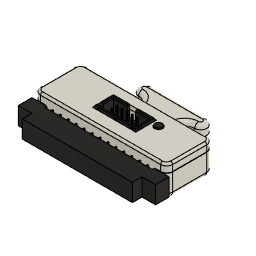
SpeedDOS_ParUP v5 (Autodesk Fusion 360 design; units mm, degrees)
Autodesk Fusion 360 part; units mm, degrees
sketch "UP-PAR-Adaptor" plane through (0, 0, 0) normal (0, 0, 1) x (1, 0, 0) in component "PCB"
  line L0 (54, 20) -> (0, 20)
  line L1 (0, 0) -> (54, 0)
  line L2 (54, 0) -> (54, 20)
  line L3 (0, 20) -> (0, 0)
  line L4 (1.3215, 4.5593) -> (1.3215, 2.9337)
  line L5 (2.4331, 2.9337) -> (3.3362, 2.9337)
  arc A0 (3.3362, 4.1529) -> (2.9298, 4.5593) centre (2.9298, 4.1529) ccw
  arc A1 (2.9298, 4.5593) -> (2.4331, 4.1981) centre (2.9298, 4.0372) ccw
  line L6 (0.87, 4.1981) -> (1.3215, 4.5593)
  line L7 (0.87, 2.9337) -> (1.7731, 2.9337)
  arc A2 (3.2007, 3.8368) -> (3.3362, 4.1529) centre (2.8997, 4.1529) ccw
  line L8 (3.2007, 3.8368) -> (2.4331, 2.9337)
  line L9 (39.6875, 9.2075) -> (39.6875, 6.6675)
  line L10 (43.09, -1) -> (43.09, 0)
  line L11 (46.55, 0) -> (46.55, -1)
  line L12 (51.01, -1) -> (51.01, 0)
  line L13 (13.97, 8.89) -> (16.51, 8.89)
  line L14 (51.01, 0) -> (50.51, 0)
  circle A3 centre (5, 15) radius 3.1789
  line L15 (50.51, 0) -> (50.51, -1)
  line L16 (39.6875, 9.2075) -> (44.7675, 9.2075)
  line L17 (45.82, 0.1) -> (45.82, -1)
  line L18 (16.51, 13.97) -> (16.51, 8.89)
  line L19 (16.51, 13.97) -> (13.97, 13.97)
  line L20 (43.09, 0) -> (42.59, 0)
  circle A4 centre (5, 15) radius 1.7463
  circle A5 centre (49, 15) radius 3.1789
  line L21 (44.7675, 6.6675) -> (39.6875, 6.6675)
  circle A6 centre (49, 15) radius 1.7463
  line L22 (49.78, 0.1) -> (49.78, -1)
  line L23 (43.82, 0.1) -> (43.82, -1)
  line L24 (7.45, -1) -> (7.45, 0)
  line L25 (3.49, 0) -> (2.99, 0)
  line L26 (37.9, 0.1) -> (37.9, -1)
  line L27 (24.02, 0.1) -> (24.02, -1)
  line L28 (34.67, 0) -> (34.67, -1)
  line L29 (22.79, 0) -> (22.79, -1)
  line L30 (13.97, 8.89) -> (13.97, 13.97)
  line L31 (44.7675, 6.6675) -> (44.7675, 9.2075)
  line L32 (23.29, 0) -> (22.79, 0)
  line L33 (29.98, 0.1) -> (29.98, -1)
  line L34 (38.63, 0) -> (38.63, -1)
  line L35 (35.17, -1) -> (35.17, 0)
  line L36 (27.25, 0) -> (26.75, 0)
  line L37 (26.75, 0) -> (26.75, -1)
  line L38 (35.17, 0) -> (34.67, 0)
  line L39 (47.05, -1) -> (47.05, 0)
  line L40 (33.94, 0.1) -> (33.94, -1)
  line L41 (23.29, -1) -> (23.29, 0)
  line L42 (47.05, 0) -> (46.55, 0)
  line L43 (27.98, 0.1) -> (27.98, -1)
  line L44 (42.59, 0) -> (42.59, -1)
  line L45 (41.86, 0.1) -> (41.86, -1)
  line L46 (35.9, 0.1) -> (35.9, -1)
  line L47 (30.71, 0) -> (30.71, -1)
  line L48 (27.25, -1) -> (27.25, 0)
  line L49 (31.94, 0.1) -> (31.94, -1)
  line L50 (39.86, 0.1) -> (39.86, -1)
  line L51 (26.02, 0.1) -> (26.02, -1)
  line L52 (39.13, 0) -> (38.63, 0)
  line L53 (47.78, 0.1) -> (47.78, -1)
  line L54 (31.21, 0) -> (30.71, 0)
  line L55 (10.18, 0.1) -> (10.18, -1)
  line L56 (7.45, 0) -> (6.95, 0)
  line L57 (8.18, 0.1) -> (8.18, -1)
  line L58 (6.22, 0.1) -> (6.22, -1)
  line L59 (4.22, 0.1) -> (4.22, -1)
  line L60 (3.49, -1) -> (3.49, 0)
  line L61 (39.13, -1) -> (39.13, 0)
  line L62 (31.21, -1) -> (31.21, 0)
  line L63 (53.8, -1) -> (0.2, -1)
  line L64 (6.95, 0) -> (6.95, -1)
  line L65 (0.2, -1) -> (0.2, 0)
  line L66 (0.2, 0) -> (-2.3, 0)
  line L67 (14.14, 0.1) -> (14.14, -1)
  line L68 (2.99, 0) -> (2.99, -1)
  line L69 (-7.25, 0) -> (-7.25, -6.8)
  line L70 (-2.3, 0) -> (-4, 0)
  line L71 (61.25, 0) -> (61.25, -6.8)
  line L72 (58, 0) -> (56.3, 0)
  line L73 (59.7, 0) -> (58, 0)
  line L74 (18.83, 0) -> (18.83, -1)
  line L75 (14.87, 0) -> (14.87, -1)
  line L76 (20.06, 0.1) -> (20.06, -1)
  line L77 (22.06, 0.1) -> (22.06, -1)
  line L78 (19.33, -1) -> (19.33, 0)
  line L79 (56.3, -1.6) -> (56.3, 0)
  line L80 (35.89, 15.3338) -> (35.89, 10.2537)
  line L81 (18.1, 0.1) -> (18.1, -1)
  line L82 (37.16, 8.825) -> (37.16, 7.3962)
  line L83 (16.84, 8.825) -> (16.84, 10.2537)
  line L84 (-4, 0) -> (-5.7, 0)
  line L85 (56.3, -6.8) -> (56.3, -5.2)
  line L86 (-2.3, -1.6) -> (-2.3, 0)
  line L87 (37.16, 7.3962) -> (16.84, 7.3962)
  line L88 (-5.7, -4.2) -> (-5.7, -2.6)
  line L89 (58, -7.2333) -> (58, -4.3667)
  line L90 (16.84, 7.3962) -> (16.84, 8.825)
  line L91 (16.1, 0.1) -> (16.1, -1)
  line L92 (-4, -8.7333) -> (-4, -11.6)
  line L93 (-5.7, -6.8) -> (-7.25, -6.8)
  line L94 (15.37, -1) -> (15.37, 0)
  line L95 (19.33, 0) -> (18.83, 0)
  line L96 (58, -8.052) -> (58, -7.9147)
  line L97 (-2.3, -4.2) -> (-2.3, -2.6)
  line L98 (-5.7, -6.8) -> (-5.7, -5.2)
  line L99 (18.11, 10.2537) -> (18.11, 15.3338)
  line L100 (12.14, 0.1) -> (12.14, -1)
  line L101 (59.7, -1.6) -> (59.7, 0)
  line L102 (15.37, 0) -> (14.87, 0)
  line L103 (29.0638, 16.6038) -> (37.16, 16.6038)
  line L104 (18.11, 15.3338) -> (24.9362, 15.3338)
  line L105 (16.84, 10.2537) -> (16.84, 16.6038)
  line L106 (-2.3, -6.8) -> (-2.3, -5.2)
  line L107 (10.91, 0) -> (10.91, -1)
  line L108 (24.9362, 16.6038) -> (29.0638, 16.6038)
  line L109 (11.41, -1) -> (11.41, 0)
  line L110 (24.9362, 15.3338) -> (29.0638, 15.3338)
  line L111 (56.3, -6.8) -> (54.5, -6.8)
  line L112 (11.41, 0) -> (10.91, 0)
  line L113 (-4, -4.3667) -> (-4, -7.2333)
  line L114 (59.7, -6.8) -> (59.7, -5.2)
  line L115 (37.16, 10.2537) -> (37.16, 8.825)
  line L116 (56.3, -4.2) -> (56.3, -2.6)
  line L117 (16.84, 16.6038) -> (24.9362, 16.6038)
  line L118 (-2.3, -6.8) -> (-5.7, -6.8)
  line L119 (54.5, -11.6) -> (-0.5, -11.6)
  line L120 (35.89, 8.6662) -> (18.11, 8.6662)
  line L121 (29.0638, 15.3338) -> (35.89, 15.3338)
  line L122 (35.89, 8.825) -> (35.89, 8.6662)
  line L123 (58, -2.8667) -> (58, 0)
  line L124 (-4, -3.548) -> (-4, -3.6853)
  line L125 (58, -3.6853) -> (58, -3.548)
  line L126 (-5.7, -1.6) -> (-5.7, 0)
  line L127 (17.6337, 10.2537) -> (16.84, 10.2537)
  line L128 (59.7, -4.2) -> (59.7, -2.6)
  line L129 (-4, -7.9147) -> (-4, -8.052)
  line L130 (58, -11.6) -> (58, -8.7333)
  line L131 (32.08, 14.6987) -> (32.3975, 15.0162)
  line L132 (61.25, 0) -> (59.7, 0)
  line L133 (36.3663, 8.19) -> (17.6337, 8.19)
  line L134 (36.3663, 8.19) -> (35.89, 8.6662)
  line L135 (35.89, 8.825) -> (36.3663, 8.825)
  line L136 (35.89, 10.2537) -> (36.3663, 10.2537)
  arc A7 (26.5238, 7.3962) -> (27.635, 7.3962) centre (27.0794, 7.3962) ccw
  line L137 (18.11, 8.6662) -> (17.6337, 8.19)
  line L138 (59.7, -6.8) -> (56.3, -6.8)
  line L139 (53.8, 0) -> (53.8, -1)
  line L140 (32.715, 15.0162) -> (32.5563, 15.0162)
  line L141 (32.5563, 15.0162) -> (32.3975, 15.0162)
  line L142 (31.9213, 15.0162) -> (32.08, 14.8575)
  line L143 (36.3663, 8.825) -> (37.16, 8.825)
  line L144 (36.3663, 8.19) -> (36.3663, 8.825)
  line L145 (24.9362, 15.3338) -> (24.9362, 15.81)
  line L146 (31.9213, 15.0162) -> (31.7625, 15.0162)
  line L147 (56.3, 0) -> (53.8, 0)
  line L148 (-4, 0) -> (-4, -2.8667)
  line L149 (24.9362, 15.81) -> (24.9362, 16.6038)
  line L150 (31.7625, 15.0162) -> (32.08, 14.6987)
  line L151 (18.11, 10.2537) -> (17.6337, 10.2537)
  line L152 (31.7625, 15.0162) -> (31.6038, 15.0162)
  line L153 (29.0638, 15.81) -> (36.3663, 15.81)
  line L154 (32.08, 14.54) -> (32.5563, 15.0162)
  line L155 (29.0638, 15.3338) -> (29.0638, 15.81)
  line L156 (18.11, 8.825) -> (18.11, 10.2537)
  line L157 (54.5, -6.8) -> (54.5, -11.6)
  line L158 (31.6038, 15.0162) -> (32.08, 14.54)
  line L159 (31.445, 15.0162) -> (32.08, 14.3812)
  line L160 (36.3663, 15.81) -> (35.89, 15.3338)
  line L161 (35.89, 10.2537) -> (35.89, 8.825)
  line L162 (-5.7, 0) -> (-7.25, 0)
  line L163 (18.11, 15.3338) -> (17.6337, 15.81)
  line L164 (-0.5, -11.6) -> (-0.5, -6.8)
  line L165 (17.6337, 8.825) -> (16.84, 8.825)
  arc A8 (18.11, 7.3962) -> (19.38, 7.3962) centre (18.745, 7.3962) ccw
  arc A9 (34.62, 7.3962) -> (35.89, 7.3962) centre (35.255, 7.3962) ccw
  line L166 (29.0638, 15.81) -> (29.0638, 16.6038)
  line L167 (-0.5, -6.8) -> (-2.3, -6.8)
  line L168 (32.08, 14.8575) -> (32.2388, 15.0162)
  line L169 (32.2388, 15.0162) -> (31.9213, 15.0162)
  line L170 (61.25, -6.8) -> (59.7, -6.8)
  line L171 (18.11, 8.6662) -> (18.11, 8.825)
  line L172 (37.16, 16.6038) -> (37.16, 10.2537)
  line L173 (31.6038, 15.0162) -> (31.445, 15.0162)
  arc A10 (39.25, 12.55) -> (38.45, 12.55) centre (38.85, 12.85) ccw
  arc A11 (38.45, 17.45) -> (39.2, 17.5) centre (38.8467, 17.1498) ccw
  line L174 (17.6337, 10.2537) -> (17.6337, 15.81)
  circle A12 centre (41, 15) radius 1.75
  line L175 (32.08, 14.3812) -> (32.715, 15.0162)
  line L176 (32.3975, 15.0162) -> (32.2388, 15.0162)
  line L177 (42.45, 12) -> (39.6, 12)
  line L178 (39.55, 18) -> (42.45, 18)
  arc A13 (43.55, 12.55) -> (42.8, 12.5) centre (43.1533, 12.8502) ccw
  line L179 (36.3663, 10.2537) -> (36.3663, 15.81)
  line L180 (18.11, 8.825) -> (17.6337, 8.825)
  line L181 (44, 17.75) -> (44, 12.25)
  arc A14 (42.75, 17.45) -> (43.5, 17.5) centre (43.1467, 17.1498) ccw
  line L182 (36.3663, 10.2537) -> (37.16, 10.2537)
  circle A15 centre (41, 15) radius 1.4
  line L183 (38, 12.6) -> (38, 17.75)
  line L184 (24.9362, 15.81) -> (17.6337, 15.81)
  line L185 (17.6337, 8.825) -> (17.6337, 8.19)
  line L186 (49.78, 0.1) -> (49.78, 4)
  line L187 (49.28, 3) -> (49.28, 2)
  arc A16 (44.32, 2) -> (45.32, 2) centre (44.82, 2) ccw
  line L188 (45.82, 0.1) -> (45.82, 4)
  line L189 (45.32, 3) -> (45.32, 2)
  arc A17 (45.32, 3) -> (44.32, 3) centre (44.82, 3) ccw
  arc A18 (49.78, 4) -> (47.78, 4) centre (48.78, 4) ccw
  arc A19 (49.28, 3) -> (48.28, 3) centre (48.78, 3) ccw
  line L190 (47.78, 0.1) -> (47.78, 4)
  arc A20 (45.82, 4) -> (43.82, 4) centre (44.82, 4) ccw
  line L191 (44.32, 3) -> (44.32, 2)
  line L192 (20.56, 3) -> (20.56, 2)
  arc A21 (17.6, 3) -> (16.6, 3) centre (17.1, 3) ccw
  line L193 (41.86, 0.1) -> (41.86, 4)
  arc A22 (33.44, 3) -> (32.44, 3) centre (32.94, 3) ccw
  line L194 (13.64, 3) -> (13.64, 2)
  arc A23 (6.22, 4) -> (4.22, 4) centre (5.22, 4) ccw
  line L195 (12.14, 0.1) -> (12.14, 4)
  arc A24 (5.72, 3) -> (4.72, 3) centre (5.22, 3) ccw
  arc A25 (26.02, 4) -> (24.02, 4) centre (25.02, 4) ccw
  arc A26 (36.4, 2) -> (37.4, 2) centre (36.9, 2) ccw
  arc A27 (48.28, 2) -> (49.28, 2) centre (48.78, 2) ccw
  arc A28 (24.52, 2) -> (25.52, 2) centre (25.02, 2) ccw
  line L196 (39.86, 0.1) -> (39.86, 4)
  arc A29 (28.48, 2) -> (29.48, 2) centre (28.98, 2) ccw
  arc A30 (16.6, 2) -> (17.6, 2) centre (17.1, 2) ccw
  arc A31 (10.18, 4) -> (8.18, 4) centre (9.18, 4) ccw
  line L197 (24.52, 3) -> (24.52, 2)
  arc A32 (18.1, 4) -> (16.1, 4) centre (17.1, 4) ccw
  arc A33 (13.64, 3) -> (12.64, 3) centre (13.14, 3) ccw
  arc A34 (9.68, 3) -> (8.68, 3) centre (9.18, 3) ccw
  arc A35 (33.94, 4) -> (31.94, 4) centre (32.94, 4) ccw
  arc A36 (41.86, 4) -> (39.86, 4) centre (40.86, 4) ccw
  line L198 (33.94, 0.1) -> (33.94, 4)
  arc A37 (20.56, 2) -> (21.56, 2) centre (21.06, 2) ccw
  line L199 (35.9, 0.1) -> (35.9, 4)
  line L200 (29.98, 0.1) -> (29.98, 4)
  line L201 (33.44, 3) -> (33.44, 2)
  line L202 (41.36, 3) -> (41.36, 2)
  arc A38 (4.72, 2) -> (5.72, 2) centre (5.22, 2) ccw
  line L203 (5.72, 3) -> (5.72, 2)
  line L204 (9.68, 3) -> (9.68, 2)
  line L205 (21.56, 3) -> (21.56, 2)
  line L206 (36.4, 3) -> (36.4, 2)
  line L207 (12.64, 3) -> (12.64, 2)
  line L208 (4.22, 0.1) -> (4.22, 4)
  line L209 (48.28, 3) -> (48.28, 2)
  arc A39 (8.68, 2) -> (9.68, 2) centre (9.18, 2) ccw
  line L210 (17.6, 3) -> (17.6, 2)
  arc A40 (22.06, 4) -> (20.06, 4) centre (21.06, 4) ccw
  arc A41 (41.36, 3) -> (40.36, 3) centre (40.86, 3) ccw
  line L211 (37.9, 0.1) -> (37.9, 4)
  line L212 (32.44, 3) -> (32.44, 2)
  line L213 (31.94, 0.1) -> (31.94, 4)
  line L214 (4.72, 3) -> (4.72, 2)
  arc A42 (37.4, 3) -> (36.4, 3) centre (36.9, 3) ccw
  arc A43 (29.48, 3) -> (28.48, 3) centre (28.98, 3) ccw
  line L215 (16.6, 3) -> (16.6, 2)
  line L216 (20.06, 0.1) -> (20.06, 4)
  arc A44 (40.36, 2) -> (41.36, 2) centre (40.86, 2) ccw
  line L217 (27.98, 0.1) -> (27.98, 4)
  line L218 (26.02, 0.1) -> (26.02, 4)
  line L219 (24.02, 0.1) -> (24.02, 4)
  line L220 (28.48, 3) -> (28.48, 2)
  arc A45 (29.98, 4) -> (27.98, 4) centre (28.98, 4) ccw
  arc A46 (37.9, 4) -> (35.9, 4) centre (36.9, 4) ccw
  line L221 (29.48, 3) -> (29.48, 2)
  line L222 (6.22, 0.1) -> (6.22, 4)
  line L223 (43.82, 0.1) -> (43.82, 4)
  arc A47 (25.52, 3) -> (24.52, 3) centre (25.02, 3) ccw
  arc A48 (32.44, 2) -> (33.44, 2) centre (32.94, 2) ccw
  line L224 (25.52, 3) -> (25.52, 2)
  line L225 (22.06, 0.1) -> (22.06, 4)
  line L226 (37.4, 3) -> (37.4, 2)
  line L227 (40.36, 3) -> (40.36, 2)
  line L228 (38, 12.2) -> (38, 12.6)
  line L229 (24.206, 13.016) -> (24.714, 13.016)
  line L230 (31.826, 10.984) -> (31.826, 10.476)
  line L231 (31.826, 10.476) -> (32.334, 10.476)
  line L232 (31.826, 13.016) -> (32.334, 13.016)
  line L233 (32.334, 13.016) -> (32.334, 13.524)
  arc A49 (43.5, 17.5) -> (42.75, 17.45) centre (43.1467, 17.1498) ccw
  line L234 (24.714, 13.524) -> (24.206, 13.524)
  line L235 (29.286, 10.476) -> (29.794, 10.476)
  line L236 (29.286, 13.524) -> (29.286, 13.016)
  line L237 (31.826, 13.524) -> (31.826, 13.016)
  line L238 (24.206, 10.984) -> (24.206, 10.476)
  arc A50 (43.8, 12) -> (44, 12.2) centre (43.8, 12.2) ccw
  line L239 (26.746, 10.476) -> (27.254, 10.476)
  line L240 (26.746, 13.524) -> (26.746, 13.016)
  line L241 (29.794, 10.984) -> (29.286, 10.984)
  line L242 (42.9, 18.5) -> (42.9, 18)
  line L243 (14.14, 0.1) -> (14.14, 4)
  arc A51 (38.2, 18) -> (38, 17.8) centre (38.2, 17.8) ccw
  line L244 (21.666, 13.016) -> (22.174, 13.016)
  line L245 (38.2, 18) -> (39.55, 18)
  line L246 (21.666, 13.524) -> (21.666, 13.016)
  line L247 (21.666, 10.476) -> (22.174, 10.476)
  line L248 (8.18, 0.1) -> (8.18, 4)
  line L249 (38, 17.75) -> (38, 17.8)
  line L250 (44, 17.8) -> (44, 17.75)
  line L251 (22.174, 13.016) -> (22.174, 13.524)
  line L252 (43.8, 12) -> (42.45, 12)
  arc A52 (42.8, 12.5) -> (43.55, 12.55) centre (43.1533, 12.8502) ccw
  line L253 (27.254, 10.476) -> (27.254, 10.984)
  line L254 (29.794, 13.524) -> (29.286, 13.524)
  line L255 (24.714, 10.984) -> (24.206, 10.984)
  line L256 (24.206, 13.524) -> (24.206, 13.016)
  line L257 (39.6, 12) -> (38.2, 12)
  line L258 (42.45, 18) -> (43.8, 18)
  line L259 (29.794, 13.016) -> (29.794, 13.524)
  line L260 (10.18, 0.1) -> (10.18, 4)
  line L261 (16.1, 0.1) -> (16.1, 4)
  line L262 (32.334, 10.984) -> (31.826, 10.984)
  line L263 (29.286, 10.984) -> (29.286, 10.476)
  arc A53 (12.64, 2) -> (13.64, 2) centre (13.14, 2) ccw
  line L264 (29.794, 10.476) -> (29.794, 10.984)
  line L265 (29.286, 13.016) -> (29.794, 13.016)
  line L266 (8.68, 3) -> (8.68, 2)
  line L267 (32.334, 13.524) -> (31.826, 13.524)
  line L268 (24.714, 13.016) -> (24.714, 13.524)
  arc A54 (39.2, 17.5) -> (38.45, 17.45) centre (38.8467, 17.1498) ccw
  arc A55 (14.14, 4) -> (12.14, 4) centre (13.14, 4) ccw
  line L269 (27.254, 10.984) -> (26.746, 10.984)
  line L270 (42.9, 18) -> (43.6, 18)
  line L271 (24.206, 10.476) -> (24.714, 10.476)
  line L272 (18.1, 0.1) -> (18.1, 4)
  line L273 (44, 12.25) -> (44, 12.2)
  line L274 (26.746, 13.016) -> (27.254, 13.016)
  line L275 (22.174, 10.984) -> (21.666, 10.984)
  line L276 (21.666, 10.984) -> (21.666, 10.476)
  line L277 (26.746, 10.984) -> (26.746, 10.476)
  line L278 (22.174, 10.476) -> (22.174, 10.984)
  arc A56 (44, 17.8) -> (43.8, 18) centre (43.8, 17.8) ccw
  line L279 (24.714, 10.476) -> (24.714, 10.984)
  line L280 (27.254, 13.524) -> (26.746, 13.524)
  arc A57 (38.45, 12.55) -> (39.25, 12.55) centre (38.85, 12.85) ccw
  line L281 (32.334, 10.476) -> (32.334, 10.984)
  arc A58 (21.56, 3) -> (20.56, 3) centre (21.06, 3) ccw
  line L282 (43.6, 11.5) -> (43.6, 12)
  line L283 (27.254, 13.016) -> (27.254, 13.524)
  line L284 (39.1, 12) -> (38.4, 12)
  line L285 (43.6, 12) -> (42.9, 12)
  arc A59 (38, 12.2) -> (38.2, 12) centre (38.2, 12.2) ccw
  line L286 (38.4, 18.5) -> (38.4, 18)
  line L287 (39.1, 18) -> (39.1, 18.5)
  line L288 (42.9, 11.5) -> (43.6, 11.5)
  line L289 (43.6, 18) -> (43.6, 18.5)
  line L290 (39.1, 11.5) -> (39.1, 12)
  line L291 (43.6, 18.5) -> (42.9, 18.5)
  line L292 (38.4, 18) -> (39.1, 18)
  line L293 (42.9, 12) -> (42.9, 11.5)
  line L294 (39.1, 18.5) -> (38.4, 18.5)
  line L295 (38.4, 11.5) -> (39.1, 11.5)
  line L296 (38.4, 12) -> (38.4, 11.5)
  line L297 (22.174, 13.524) -> (21.666, 13.524)
extrude "Extrude1" add sketch "UP-PAR-Adaptor" against normal blind 1.6 contours L0 L1 L2 L3 L14 L17 L20 L22 L23 L25 L26 L27 L32 L33 L36 L38 L40 L42 L43 L45 L46 L49 L50 L51 L52 L53 L54 L55 L56 L57 L58 L59 L66 L67 L76 L77 L81 L91 L95 L100 L102 L112 L147 L186 L188 A18 L190 A20 L193 A23 L195 A25 L196 A31 A32 A35 A36 L198 L199 L200 L208 A40 L211 L213 L216 L217 L218 L219 A45 A46 L222 L223 L225 L243 L248 L260 L261 A55 L272 | L1 L22 L53 L186 A18 L190 | L1 L58 L59 A23 L208 L222 | L1 L17 L23 L188 A20 L223 | L1 L55 L57 A31 L248 L260 | L1 L45 L50 L193 L196 A36 | L1 L67 L100 L195 L243 A55 | L1 L26 L46 L199 L211 A46 | L1 L81 L91 A32 L261 L272 | L1 L40 L49 A35 L198 L213 | L1 L76 L77 A40 L216 L225 | L1 L33 L43 L200 L217 A45 | L1 L27 L51 A25 L218 L219 | L9 L16 L21 L31 | L13 L18 L19 L30 | A3 | A5 | L80 L136 L160 L179 | L80 L99 L104 L110 L120 L121 L122 L156 L161 L171 | L121 L153 L155 L160 | L115 L135 L136 L143 L161 L182 | L108 L110 L145 L149 L155 L166 | L103 L153 L166 L172 L179 L182 | L122 L134 L135 L144 | L104 L145 L163 L184 | L120 L133 L134 L137 | L82 L87 L90 L133 L143 L144 L165 L185 | L99 L151 L163 L174 | L105 L117 L127 L149 L174 L184 | L137 L171 L180 L185 | L83 L127 L151 L156 L165 L180 | L87 A9 | L87 A7 | L87 A8 | L131 L142 L146 L150 L168 L176 | L131 L141 L150 L152 L154 L158 | L140 L154 L158 L159 L173 L175 | L142 L168 L169 | A10 A57 | A11 A54 | A12 | L177 L178 L181 L183 L228 A50 A51 L245 L249 L250 L252 L257 L258 L270 L273 A56 L284 L285 A59 L292 | L252 L282 L285 L288 L293 | L257 L284 L290 L295 L296 | L242 L258 L270 L289 L291 | L245 L286 L287 L292 L294 | A13 A52 | A14 A49 | A15 | L187 A19 A27 L209 | A16 L189 A17 L191 | L192 A37 L205 A58 | A21 A30 L210 L215 | A22 L201 L212 A48 | L194 A33 L207 A53 | A24 A38 L203 L214 | A26 L206 A42 L226 | A28 L197 A47 L224 | A29 A43 L220 L221 | A34 L204 A39 L266 | L202 A41 A44 L227 | L229 L234 L256 L268 | L230 L231 L262 L281 | L232 L233 L237 L267 | L235 L241 L263 L264 | L236 L254 L259 L265 | L238 L255 L271 L279 | L239 L253 L269 L277 | L240 L274 L280 L283 | L244 L246 L251 L297 | L247 L275 L276 L278 makes body 1 in component "PCB"
extrude "Extrude2" add sketch "UP-PAR-Adaptor" along normal blind 3 contours L177 L178 L181 L183 L228 A50 A51 L245 L249 L250 L252 L257 L258 L270 L273 A56 L284 L285 A59 L292 bodies 1 in component "PCB"
extrude "Extrude3" add sketch "UP-PAR-Adaptor" along normal blind 3.8 contours A10 A57 | A11 A54 | A13 A52 | A14 A49 bodies 1 in component "PCB"
extrude "Extrude4" add sketch "UP-PAR-Adaptor" along normal blind 9 contours A12 | A15 bodies 1 in component "PCB"
extrude "Extrude5" add sketch "UP-PAR-Adaptor" along normal blind 2.3 contours L80 L99 L104 L110 L120 L121 L122 L156 L161 L171 | L115 L135 L136 L143 L161 L182 | L108 L110 L145 L149 L155 L166 | L83 L127 L151 L156 L165 L180 bodies 1 in component "PCB"
extrude "Extrude6" add sketch "UP-PAR-Adaptor" along normal blind 9.3 contours L80 L136 L160 L179 | L121 L153 L155 L160 | L103 L153 L166 L172 L179 L182 | L122 L134 L135 L144 | L104 L145 L163 L184 | L120 L133 L134 L137 | L82 L87 L90 L133 L143 L144 L165 L185 | L99 L151 L163 L174 | L105 L117 L127 L149 L174 L184 | L137 L171 L180 L185 bodies 1 in component "PCB"
extrude "Extrude7" add sketch "UP-PAR-Adaptor" along normal blind 8.8 contours L229 L234 L256 L268 | L230 L231 L262 L281 | L232 L233 L237 L267 | L235 L241 L263 L264 | L236 L254 L259 L265 | L238 L255 L271 L279 | L239 L253 L269 L277 | L240 L274 L280 L283 | L244 L246 L251 L297 | L247 L275 L276 L278 bodies 1 in component "PCB"
extrude "Extrude8" add sketch "UP-PAR-Adaptor" along normal blind 8.8 contours L87 A9 | L87 A7 | L87 A8 bodies 1 in component "PCB"
extrude "Extrude9" add sketch "UP-PAR-Adaptor" along normal blind 4.3 and the other way blind 4.4 contours L1 L63 L65 L66 L69 L70 L71 L72 L73 L84 L93 L111 L118 L119 L132 L138 L139 L147 L157 L162 L164 L167 L170 | L1 L12 L14 L15 L63 | L1 L25 L60 L63 L68 | L1 L11 L39 L42 L63 | L1 L24 L56 L63 L64 | L1 L10 L20 L44 L63 | L1 L63 L107 L109 L112 | L1 L34 L52 L61 L63 | L1 L63 L75 L94 L102 | L1 L28 L35 L38 L63 | L1 L63 L74 L78 L95 | L1 L47 L54 L62 L63 | L1 L29 L32 L41 L63 | L1 L36 L37 L48 L63 bodies 1 in component "PCB"
extrude "Extrude10" add sketch "UP-PAR-Adaptor" along normal blind 0.5 contours L1 L22 L53 L63 | L1 L22 L53 L186 A18 L190 | L1 L58 L59 A23 L208 L222 | L1 L58 L59 L63 | L1 L17 L23 L63 | L1 L17 L23 L188 A20 L223 | L1 L55 L57 A31 L248 L260 | L1 L55 L57 L63 | L1 L45 L50 L63 | L1 L45 L50 L193 L196 A36 | L1 L67 L100 L195 L243 A55 | L1 L63 L67 L100 | L1 L26 L46 L63 | L1 L26 L46 L199 L211 A46 | L1 L81 L91 A32 L261 L272 | L1 L63 L81 L91 | L1 L40 L49 L63 | L1 L40 L49 A35 L198 L213 | L1 L76 L77 A40 L216 L225 | L1 L63 L76 L77 | L1 L33 L43 L63 | L1 L33 L43 L200 L217 A45 | L1 L27 L51 A25 L218 L219 | L1 L27 L51 L63 bodies 1 in component "PCB"
extrude "Extrude11" add sketch "UP-PAR-Adaptor" against normal blind 0.5 from surface at -1.6 contours L1 L22 L53 L63 | L1 L22 L53 L186 A18 L190 | L1 L58 L59 A23 L208 L222 | L1 L58 L59 L63 | L1 L17 L23 L63 | L1 L17 L23 L188 A20 L223 | L1 L55 L57 A31 L248 L260 | L1 L55 L57 L63 | L1 L45 L50 L63 | L1 L45 L50 L193 L196 A36 | L1 L67 L100 L195 L243 A55 | L1 L63 L67 L100 | L1 L26 L46 L63 | L1 L26 L46 L199 L211 A46 | L1 L81 L91 A32 L261 L272 | L1 L63 L81 L91 | L1 L40 L49 L63 | L1 L40 L49 A35 L198 L213 | L1 L76 L77 A40 L216 L225 | L1 L63 L76 L77 | L1 L33 L43 L63 | L1 L33 L43 L200 L217 A45 | L1 L27 L51 A25 L218 L219 | L1 L27 L51 L63 bodies 1 in component "PCB"
chamfer "Chamfer1" distance 0.5 angle 45 7 edges at (27, 8.6662, 9.3) (35.89, 12.7938, 9.3) (32.4769, 15.3338, 9.3) (21.5231, 15.3338, 9.3) (18.11, 12.7938, 9.3) (18.11, 8.7456, 9.3) (35.89, 8.7456, 9.3) on bodies 1 in component "PCB"
ref_plane "WorkPlane1" through (0, 0, -4.4) normal (0, 0, 1) x (1, 0, 0) in component "bottom_shell"
sketch "bottom" plane through (0, 0, -4.4) normal (0, 0, 1) x (1, 0, 0) in component "bottom_shell"
  circle A0 centre (49, 15) radius 1.7463 construction
  line L0 (54, 0) -> (54, 20) construction
  line L1 (54, 20) -> (0, 20) construction
  line L2 (0, 20) -> (0, 0) construction
  circle A1 centre (5, 15) radius 1.7463 construction
  line L3 (27, 20) -> (27, -5) construction
  line L4 (54, 0) -> (0, 0) construction
  circle A2 centre (49, 15) radius 1.75
  circle A3 centre (5, 15) radius 1.75
  line L5 (60, 3) -> (60, 20)
  line L6 (-6, 3) -> (-6, 20)
  line L7 (57, 23) -> (-3, 23)
  line L8 (57, 0) -> (-3, 0)
  arc A4 (57, 0) -> (60, 3) centre (57, 3) ccw
  arc A5 (60, 20) -> (57, 23) centre (57, 20) ccw
  arc A6 (-3, 23) -> (-6, 20) centre (-3, 20) ccw
  arc A7 (-6, 3) -> (-3, 0) centre (-3, 3) ccw
  line L9 (57, 21) -> (-3, 21)
  arc A8 (-3, 21) -> (-4, 20) centre (-3, 20) ccw
  line L10 (-4, 3) -> (-4, 20)
  arc A9 (-4, 3) -> (-3, 2) centre (-3, 3) ccw
  line L11 (57, 2) -> (-3, 2)
  arc A10 (57, 2) -> (58, 3) centre (57, 3) ccw
  line L12 (58, 3) -> (58, 20)
  arc A11 (58, 20) -> (57, 21) centre (57, 20) ccw
  circle A12 centre (49, 15) radius 4.25
  circle A13 centre (5, 15) radius 4.25
  line L13 (54.6, 1.2) -> (54.6, 2)
  line L14 (-0.6, 0) -> (-0.6, 2)
  circle A14 centre (49, 15) radius 3
  circle A15 centre (5, 15) radius 3
  line L15 (57, 21.8) -> (-3, 21.8)
  arc A16 (-3, 21.8) -> (-4.8, 20) centre (-3, 20) ccw
  line L16 (-4.8, 3) -> (-4.8, 20)
  arc A17 (-4.8, 3) -> (-3, 1.2) centre (-3, 3) ccw
  arc A18 (57, 1.2) -> (58.8, 3) centre (57, 3) ccw
  line L17 (58.8, 3) -> (58.8, 20)
  arc A19 (58.8, 20) -> (57, 21.8) centre (57, 20) ccw
  line L18 (57, 1.2) -> (54.6, 1.2)
  line L19 (-0.6, 1.2) -> (-3, 1.2)
  line L20 (54.6, 1.2) -> (54.6, 0)
  line L21 (41, 28) -> (41, 33) construction
  line L22 (41, 33) -> (13, 33) construction
  line L23 (41, 33) -> (41, 39.5) construction
  line L24 (13, 39) -> (41, 39)
  line L25 (13, 36) -> (13, 39) construction
  arc A20 (13, 39) -> (13, 33) centre (13, 36) ccw
  arc A21 (41, 33) -> (41, 39) centre (41, 36) ccw
  arc A22 (41, 33) -> (41, 23) centre (41, 28) ccw
  arc A23 (13, 23) -> (13, 33) centre (13, 28) ccw
  point P0 (51.01, 0)
  point P1 (60, 0)
  point P2 (60, 23)
  point P3 (-6, 0)
  point P4 (-6, 23)
  dimension "d181" = 3.5
  dimension "d182" = 3.5
  dimension "d186" = 3
  dimension "d187" = 23
  dimension "d188" = 66
  dimension "d190" = 8.5
  dimension "d191" = 8.5
  dimension "d192" = 0.6
  dimension "d193" = 0.6
  dimension "d194" = 6
  dimension "d195" = 6
  dimension "d197" = 1.2
  dimension "d236" = 10
  dimension "d237" = 14
  dimension "d238" = 5
  dimension "d239" = 6
  constraint midpoint L1 L3.start
  constraint perpendicular L1 L3
  constraint coincident L0.start L4.start
  constraint coincident L2.end L4.end
  constraint concentric A0 A2
  constraint concentric A1 A3
  constraint vertical L5
  constraint perpendicular L4 L6
  constraint symmetric L3 L5 L6
  constraint perpendicular L5 L7
  constraint collinear L4 L8
  constraint coincident P1 L5
  constraint tangent L5 A4
  constraint tangent L8 A4
  constraint coincident P2 L5
  constraint coincident P2 L7
  constraint tangent L5 A5
  constraint tangent L7 A5
  constraint equal A4 A5
  constraint coincident P4 L6
  constraint coincident P4 L7
  constraint tangent L6 A6
  constraint tangent L7 A6
  constraint equal A4 A6
  constraint coincident P3 L6
  constraint coincident P3 L8
  constraint tangent L6 A7
  constraint tangent L8 A7
  constraint equal A4 A7
  constraint concentric A0 A12
  constraint concentric A3 A13
  constraint coincident L11 L13.end
  constraint perpendicular L11 L13
  constraint coincident L8 L14.start
  constraint coincident L11 L14.end
  constraint perpendicular L11 L14
  constraint concentric A2 A14
  constraint concentric A3 A15
  constraint parallel L7 L15
  constraint concentric A6 A16
  constraint parallel L6 L16
  constraint concentric A7 A17
  constraint parallel L8 L18
  constraint concentric A4 A18
  constraint parallel L5 L17
  constraint concentric A5 A19
  constraint tangent L15 A19
  constraint tangent A16 L16
  constraint tangent L15 A16
  constraint tangent L17 A19
  constraint tangent L16 A17
  constraint tangent A17 L18
  constraint tangent A18 L18
  constraint tangent A18 L17
  constraint collinear L18 L19
  constraint coincident L14 L19.start
  constraint coincident L8 L20.end
  constraint perpendicular L8 L20
  constraint symmetric L3 A22 A23
  constraint coincident L21.start A22.centre
  constraint vertical L21
  constraint tangent L22 A23
  constraint tangent L22 A21
  constraint perpendicular L22 L23
  constraint coincident A21.centre L23
  constraint symmetric L3 A20 A21
  constraint coincident L23 L24.end
  constraint tangent L24 A21
  constraint coincident L25.start A20.centre
  constraint perpendicular L24 L25
  constraint coincident L7 A22.end
  constraint coincident L7 A23.start
  measures "d181" diameter of A2
  measures "d182" diameter of A3
  measures "d186" radius of A4
  measures "d187" distance of L7 L8
  measures "d188" distance of L5 L6
  measures "d190" diameter of A12
  measures "d191" diameter of A13
  measures "d192" distance of L0 L13
  measures "d193" distance of L2 L14
  measures "d194" diameter of A14
  measures "d195" diameter of A15
  measures "d197" distance of L7 L15
  measures "d236" diameter of A22
  measures "d237" distance of L3 L21.start
  measures "d238" distance of L7 L21.start
  measures "d239" diameter of A21
extrude "Extrude1'" add sketch "bottom" against normal blind 2 separate body contours L5 L6 L7 L8 A4 A5 A6 A7 L14 L15 A16 L16 A17 A18 L17 A19 L18 L19 L20 | L8 L11 L13 L14 L20 | L7 L24 A20 A21 A22 A23 | L9 A8 L10 A9 L11 A10 L12 A11 L13 L14 L15 A16 L16 A17 A18 L17 A19 L18 L19 | L9 A8 L10 A9 L11 A10 L12 A11 | A12 | A13 makes body 2 in component "bottom_shell"
extrude "Extrude2'" add sketch "bottom" along normal blind 2.8 contours A12 | A13 | A14 | A15 bodies 2 in component "bottom_shell"
extrude "Extrude3'" add sketch "bottom" along normal blind 1.8 contours L8 L11 L13 L14 L20 bodies 2 in component "bottom_shell"
extrude "Extrude4'" add sketch "bottom" along normal blind 9.7 contours L9 A8 L10 A9 L11 A10 L12 A11 L13 L14 L15 A16 L16 A17 A18 L17 A19 L18 L19 bodies 2 in component "bottom_shell"
extrude "Extrude5'" add sketch "bottom" along normal blind 8.7 contours L5 L6 L7 L8 A4 A5 A6 A7 L14 L15 A16 L16 A17 A18 L17 A19 L18 L19 L20 bodies 2 in component "bottom_shell"
extrude "Extrude6'" add sketch "bottom" along normal blind 5 contours L7 L24 A20 A21 A22 A23 bodies 2 in component "bottom_shell"
fillet "Fillet1" radius 1 8 edges at (27, 2, -4.4) (57.7071, 2.2929, -4.4) (58, 11.5, -4.4) (57.7071, 20.7071, -4.4) (27, 21, -4.4) (-3.7071, 20.7071, -4.4) (-4, 11.5, -4.4) (-3.7071, 2.2929, -4.4) on bodies 2 in component "bottom_shell"
fillet "Fillet2" radius 1 2 edges at (1.0376, 16.5369, -4.4) (45.0376, 16.5369, -4.4) on bodies 2 in component "bottom_shell"
chamfer "Chamfer1'" distance 1 angle 45 2 edges at (1.0376, 13.4631, -1.6) (45.0376, 13.4631, -1.6) on bodies 2 in component "bottom_shell"
fillet "Fillet4" radius 2 20 edges at (5, 23, -6.4) (18, 28, -6.4) (10, 36, -6.4) (27, 39, -6.4) (44, 36, -6.4) (36, 28, -6.4) (49, 23, -6.4) (59.1213, 22.1213, -6.4) (60, 11.5, -6.4) (59.1213, 0.8787, -6.4) (27, 0, -6.4) (-5.1213, 0.8787, -6.4) (-6, 11.5, -6.4) (-5.1213, 22.1213, -6.4) (36, 28, 0.6) (44, 36, 0.6) (27, 39, 0.6) (10, 36, 0.6) (18, 28, 0.6) (27, 23, 0.6) on bodies 2 in component "bottom_shell"
ref_plane "WorkPlane1" through (0, 0, 6.5) normal (0, 0, 1) x (1, 0, 0) in component "top_shell"
sketch "top" plane through (0, 0, 6.5) normal (0, 0, 1) x (1, 0, 0) in component "top_shell"
  line L0 (16.84, 16.6038) -> (24.9362, 16.6038) construction
  line L1 (24.9362, 16.6038) -> (29.0638, 16.6038) construction
  line L2 (16.84, 10.2537) -> (16.84, 16.6038) construction
  line L3 (16.84, 8.825) -> (16.84, 10.2537) construction
  line L4 (16.84, 7.3962) -> (16.84, 8.825) construction
  line L5 (37.16, 7.3962) -> (16.84, 7.3962) construction
  line L6 (37.16, 8.825) -> (37.16, 7.3962) construction
  line L7 (37.16, 10.2537) -> (37.16, 8.825) construction
  line L8 (37.16, 16.6038) -> (37.16, 10.2537) construction
  line L9 (29.0638, 16.6038) -> (37.16, 16.6038) construction
  circle A0 centre (41, 15) radius 1.4 construction
  line L10 (57, 23) -> (-3, 23)
  arc A1 (-3, 23) -> (-6, 20) centre (-3, 20) ccw
  line L11 (-6, 3) -> (-6, 20)
  arc A2 (-6, 3) -> (-3, 0) centre (-3, 3) ccw
  line L12 (57, 0) -> (-3, 0)
  line L13 (57, 2) -> (-3, 2)
  arc A3 (-4, 3) -> (-3, 2) centre (-3, 3) ccw
  line L14 (-4, 3) -> (-4, 20)
  arc A4 (-3, 21) -> (-4, 20) centre (-3, 20) ccw
  line L15 (57, 21) -> (-3, 21)
  line L16 (58, 3) -> (58, 20)
  arc A5 (58, 20) -> (57, 21) centre (57, 20) ccw
  arc A6 (57, 2) -> (58, 3) centre (57, 3) ccw
  arc A7 (57, 0) -> (60, 3) centre (57, 3) ccw
  line L17 (60, 3) -> (60, 20)
  arc A8 (60, 20) -> (57, 23) centre (57, 20) ccw
  line L18 (-0.6, 0) -> (-0.6, 2)
  line L19 (54.6, 1.2) -> (54.6, 0)
  line L20 (54.6, 1.2) -> (54.6, 2)
  circle A9 centre (5, 15) radius 1.75 construction
  circle A10 centre (49, 15) radius 1.75 construction
  circle A11 centre (5, 15) radius 1.25
  circle A12 centre (49, 15) radius 1.25
  circle A13 centre (41, 15) radius 2
  line L21 (16.24, 17.2038) -> (37.76, 17.2038)
  line L22 (37.76, 17.2038) -> (37.76, 6.7962)
  line L23 (37.76, 6.7962) -> (16.24, 6.7962)
  line L24 (16.24, 6.7962) -> (16.24, 17.2038)
  circle A14 centre (5, 15) radius 3.5
  circle A15 centre (49, 15) radius 3.5
  line L25 (59.2, 3) -> (59.2, 20)
  arc A16 (59.2, 20) -> (57, 22.2) centre (57, 20) ccw
  line L26 (57, 22.2) -> (-3, 22.2)
  arc A17 (-3, 22.2) -> (-5.2, 20) centre (-3, 20) ccw
  line L27 (-5.2, 3) -> (-5.2, 20)
  arc A18 (-5.2, 3) -> (-3, 0.8) centre (-3, 3) ccw
  arc A19 (57, 0.8) -> (59.2, 3) centre (57, 3) ccw
  line L28 (57, 0.8) -> (54.6, 0.8)
  line L29 (-0.6, 0.8) -> (-3, 0.8)
  dimension "d213" = 2.5
  dimension "d214" = 2.5
  dimension "d215" = 4
  dimension "d216" = 0.6
  dimension "d217" = 0.6
  dimension "d218" = 0.6
  dimension "d219" = 0.6
  dimension "d220" = 7
  dimension "d221" = 7
  dimension "d223" = 0.8
  constraint concentric A9 A11
  constraint concentric A10 A12
  constraint concentric A0 A13
  constraint horizontal L21
  constraint vertical L22
  constraint horizontal L23
  constraint vertical L24
  constraint concentric A11 A14
  constraint concentric A12 A15
  constraint parallel L17 L25
  constraint concentric A8 A16
  constraint parallel L10 L26
  constraint concentric A1 A17
  constraint parallel L11 L27
  constraint concentric A2 A18
  constraint parallel L12 L28
  constraint concentric A7 A19
  constraint tangent L27 A18
  constraint tangent L25 A19
  constraint tangent A18 L28
  constraint tangent L25 A16
  constraint tangent A16 L26
  constraint tangent L26 A17
  constraint tangent A17 L27
  constraint tangent A19 L28
  constraint coincident L19 L28.end
  constraint coincident L18 L29.start
  constraint collinear L28 L29
  measures "d213" diameter of A11
  measures "d214" diameter of A12
  measures "d215" diameter of A13
  measures "d216" distance of L0 L21
  measures "d217" distance of L5 L23
  measures "d218" distance of L2 L24
  measures "d219" distance of L6 L22
  measures "d220" diameter of A14
  measures "d221" diameter of A15
  measures "d223" distance of L10 L26
extrude "Extrude1''" add sketch "top" along normal blind 2 separate body contours L10 A1 L11 A2 L12 A7 L17 A8 L18 L19 L25 A16 L26 A17 L27 A18 A19 L28 L29 | L12 L13 L18 L19 L20 | L13 A3 L14 A4 L15 L16 A5 A6 L18 L19 L20 L25 A16 L26 A17 L27 A18 A19 L28 L29 | L13 A3 L14 A4 L15 L16 A5 A6 | A11 | A12 | A14 | A15 makes body 3 in component "top_shell"
extrude "Extrude2''" add sketch "top" against normal blind 6.3 contours A14 | A15 bodies 3 in component "top_shell"
extrude "Extrude3''" add sketch "top" against normal blind 1 contours L13 A3 L14 A4 L15 L16 A5 A6 L18 L19 L20 L25 A16 L26 A17 L27 A18 A19 L28 L29 bodies 3 in component "top_shell"
extrude "Extrude4''" add sketch "top" against normal blind 3.5 contours L12 L13 L18 L19 L20 bodies 3 in component "top_shell"
extrude "Extrude5''" add sketch "top" against normal blind 2 contours L10 A1 L11 A2 L12 A7 L17 A8 L18 L19 L25 A16 L26 A17 L27 A18 A19 L28 L29 bodies 3 in component "top_shell"
fillet "Fillet1'" radius 1 10 edges at (27, 21, 6.5) (57.7071, 20.7071, 6.5) (58, 11.5, 6.5) (57.7071, 2.2929, 6.5) (27, 2, 6.5) (-3.7071, 2.2929, 6.5) (-4, 11.5, 6.5) (-3.7071, 20.7071, 6.5) (1.7369, 13.7343, 6.5) (45.7369, 13.7343, 6.5) on bodies 3 in component "top_shell"
fillet "Fillet2'" radius 1 8 edges at (-6, 11.5, 8.5) (-5.1213, 0.8787, 8.5) (27, 0, 8.5) (59.1213, 0.8787, 8.5) (60, 11.5, 8.5) (59.1213, 22.1213, 8.5) (27, 23, 8.5) (-5.1213, 22.1213, 8.5) on bodies 3 in component "top_shell"
component "PCB" placed x (1, 0, 0) y (0, 1, 0) z (0, 0, 1) at (0, 0, 0)
component "bottom_shell" placed x (1, 0, 0) y (0, 1, 0) z (0, 0, 1) at (0, 0, 0)
component "top_shell" placed x (1, 0, 0) y (0, 1, 0) z (0, 0, 1) at (0, 0, 0)
equation "pcb_thickness = 1.6 mm"
equation "below = 2.8 mm + pcb_thickness"
equation "wall = 2 mm"
equation "width = pcb_width + 2 mm + 2 * r_corner + 2 * wall"
equation "length = pcb_length + 1 mm + wall"
equation "above = 8.5 mm - wall"
equation "pcb_width = 54 mm"
equation "pcb_length = 20 mm"
equation "r_corner = 3 mm"
equation "drill = 3.5 mm"
equation "d_screw = 7 mm"
equation "tol_x = 0.3 mm"
equation "tol_connector = 0.6 mm"
equation "d_post = 8.5 mm"
equation "d_post2 = 8 mm"
equation "bottom_height = 4.3 mm + below"
equation "overlap = 1 mm"
equation "top_height = above + below - bottom_height - tol_y"
equation "d35 = tol_connector"
equation "d37 = d35"
equation "tol_y = 0.2 mm"
equation "d154 = -pcb_thickness"
equation "d176 = -pcb_thickness"
equation "d180 = -below"
equation "d181 = drill"
equation "d182 = drill"
equation "d186 = r_corner"
equation "d187 = length"
equation "d188 = width"
equation "d189 = -wall"
equation "d190 = d_post"
equation "d191 = d_post"
equation "d192 = tol_connector"
equation "d193 = tol_connector"
equation "d195 = d194"
equation "d197 = 0.6 * wall"
equation "d198 = -wall"
equation "d200 = below - pcb_thickness"
equation "d202 = below - pcb_thickness - 1 mm"
equation "d204 = bottom_height + overlap"
equation "d206 = bottom_height"
equation "d212 = above"
equation "d216 = tol_connector"
equation "d217 = tol_connector"
equation "d218 = tol_connector"
equation "d219 = tol_connector"
equation "d220 = d_screw"
equation "d221 = d_screw"
equation "d223 = 0.4 * wall"
equation "d224 = wall"
equation "d226 = -above + tol_y"
equation "d228 = -top_height + overlap"
equation "d230 = -top_height - 1.5 mm"
equation "d232 = -top_height"
equation "d238 = d236 / 2"
named bodies: "PCB", "bottom", "top"
